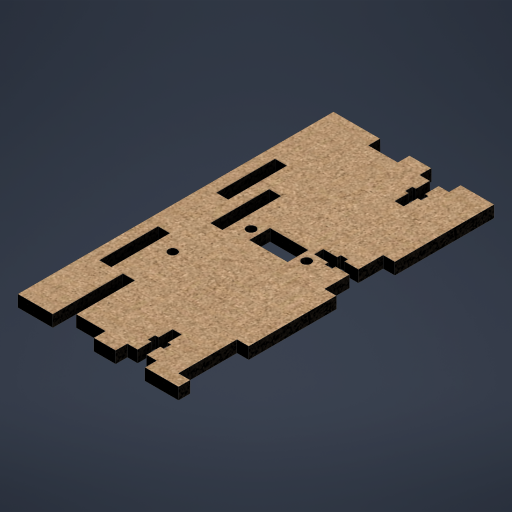
# Autodesk Inventor part: FloorButtonHolder_Top_V1_B
Saved by Autodesk Inventor 2024.1 (Build 281209000, 209)
## iProperties
Created: 2023-05-20
Part Number: FloorButtonHolder_Top_V1_B
Material: MDF Medium Density Fiberboard
Document SubType Name: Modeling
Designer: jaege
Density: 0.8 g/cm^3
Appearance: Cardboard - Corrugated
Author: jaege
Autodesk Inventor part; units mm, degrees
ref_plane "YZ Plane" through (0, 0, 0) normal (1, 0, 0) x (0, 1, 0)
ref_plane "XZ Plane" through (0, 0, 0) normal (0, 1, 0) x (-1, 0, 0)
ref_plane "XY Plane" through (0, 0, 0) normal (0, 0, 1) x (1, 0, 0)
sketch "Sketch1" plane through (0, 0, 0) normal (0, 1, 0) x (-1, 0, 0)
  line L0 (-17.5, 50) -> (17.5, 50)
  line L1 (17.5, 50) -> (17.5, -50)
  line L2 (17.5, -50) -> (-17.5, -50)
  line L3 (-17.5, -50) -> (-17.5, 50)
  line L4 (-17.5, 50) -> (17.5, -50) construction
  line L5 (17.5, 50) -> (-17.5, -50) construction
  line L6 (7.5, 50) -> (0, 50)
  line L7 (0, 50) -> (0, 54)
  line L8 (0, 54) -> (7.5, 54)
  line L9 (7.5, 54) -> (7.5, 50)
  line L10 (-10, 50) -> (-21.5, 50)
  line L11 (-21.5, 50) -> (-21.5, 54)
  line L12 (-21.5, 54) -> (-10, 54)
  line L13 (-10, 54) -> (-10, 50)
  line L14 (17.5, 30) -> (21.5, 30)
  line L15 (21.5, 30) -> (21.5, 0)
  line L16 (21.5, 0) -> (17.5, 0)
  line L17 (17.5, 0) -> (17.5, 30)
  line L18 (17.5, -20) -> (21.5, -20)
  line L19 (21.5, -20) -> (21.5, -54)
  line L20 (21.5, -54) -> (17.5, -54)
  line L21 (17.5, -54) -> (17.5, -20)
  line L22 (7.5, -50) -> (0, -50)
  line L23 (0, -50) -> (0, -54)
  line L24 (0, -54) -> (7.5, -54)
  line L25 (7.5, -54) -> (7.5, -50)
  line L26 (-10, -50) -> (-21.5, -50)
  line L27 (-21.5, -50) -> (-21.5, -54)
  line L28 (-21.5, -54) -> (-10, -54)
  line L29 (-10, -54) -> (-10, -50)
  line L30 (-17.5, 30) -> (-21.5, 30)
  line L31 (-21.5, 30) -> (-21.5, 0)
  line L32 (-21.5, 0) -> (-17.5, 0)
  line L33 (-17.5, 0) -> (-17.5, 30)
  line L34 (-17.5, -50) -> (-21.5, -50)
  line L35 (-21.5, -50) -> (-21.5, -20)
  line L36 (-21.5, -20) -> (-17.5, -20)
  line L37 (-17.5, -20) -> (-17.5, -50)
  point P0 (0, 0)
  point P1 (17.5, 0)
  point P2 (-17.5, 0)
  point P3 (-17.5, -20)
  point P4 (-21.5, -50)
  point P5 (0, -50)
  point P6 (17.5, -50)
  dimension "d0" = 35
  dimension "d2" = 7.5
  dimension "d3" = 4
  dimension "d4" = 11.5
  dimension "d5" = 4
  dimension "d6" = 10
  dimension "d7" = 10
  dimension "d8" = 4
  dimension "d9" = 30
  dimension "d10" = 4
  dimension "d11" = 34
  dimension "d12" = 20
  dimension "d13" = 20
  dimension "d14" = 7.5
  dimension "d15" = 4
  dimension "d16" = 11.5
  dimension "d17" = 4
  dimension "d18" = 10
  dimension "d19" = 10
  dimension "d20" = 4
  dimension "d21" = 30
  dimension "d22" = 20
  dimension "d23" = 4
  dimension "d24" = 30
  dimension "d27" = 4
  constraints: 76 end point, 18 parallel, 9 horizontal, 9 perpendicular, 7 point on line, 2 midpoint
  measures "d0" distance of L1.end L2.end
  measures "d2" distance of L7.end L8.end
  measures "d3" distance of L6.end L7.end
  measures "d4" distance of L11.end L12.end
  measures "d5" distance of L10.end L11.end
  measures "d6" distance between parallel lines of L9 L1
  measures "d7" distance between parallel lines of L13 L7
  measures "d8" distance of L15.end L16.end
  measures "d9" distance of L14.end L15.end
  measures "d10" distance of L19.end L20.end
  measures "d11" distance of L18.end L19.end
  measures "d12" distance between parallel lines of L16 L18
  measures "d13" distance between parallel lines of L0 L14
  measures "d14" distance of L24.end L23.end
  measures "d15" distance of L23.end L22.end
  measures "d16" distance of L28.end L27.end
  measures "d17" distance of L27.end L26.end
  measures "d18" distance between parallel lines of L25 L21
  measures "d19" distance between parallel lines of L29 L23
  measures "d20" distance of L32.end L31.end
  measures "d21" distance of L31.end L30.end
  measures "d22" distance between parallel lines of L10 L30
  measures "d23" distance of L35.end L36.end
  measures "d24" distance of L34.end L35.end
  measures "d27" distance between parallel lines of L2 L20
extrude "Extrusion1" add sketch "Sketch1" along normal blind 4
sketch "Sketch2" plane through (0, 4, 0) normal (0, 1, 0) x (1, 0, 0)
  line L0 (-21.5, 54) -> (-33.5, 54)
  line L1 (-33.5, 54) -> (-33.5, -54)
  line L2 (-33.5, -54) -> (-21.5, -54)
  line L3 (-21.5, -54) -> (-21.5, 54)
  line L4 (-7.5, -54) -> (0, -54) projected
  line L5 (-21.5, 54) -> (-21.5, 20) projected
  line L6 (-21.5, 20) -> (-17.5, 20) projected
  line L7 (-17.5, 20) -> (-17.5, 0) projected
  line L8 (-17.5, 0) -> (-21.5, 0) projected
  line L9 (-21.5, 0) -> (-21.5, -30) projected
  line L10 (-21.5, -30) -> (-17.5, -30) projected
  line L11 (-17.5, -30) -> (-17.5, -50) projected
  line L12 (-17.5, -50) -> (-7.5, -50) projected
  line L13 (-7.5, -50) -> (-7.5, -54) projected
  line L14 (-7.5, -54) -> (0, -54) projected
  line L15 (0, -54) -> (0, -50) projected
  line L16 (0, -50) -> (10, -50) projected
  line L17 (10, -50) -> (10, -54) projected
  line L18 (10, -54) -> (21.5, -54) projected
  line L19 (21.5, -54) -> (21.5, -50) projected
  line L20 (21.5, -50) -> (17.5, -50) projected
  line L21 (17.5, -50) -> (17.5, -30) projected
  line L22 (17.5, -30) -> (21.5, -30) projected
  line L23 (21.5, -30) -> (21.5, 0) projected
  line L24 (21.5, 0) -> (17.5, 0) projected
  line L25 (17.5, 0) -> (17.5, 20) projected
  line L26 (17.5, 20) -> (21.5, 20) projected
  line L27 (21.5, 20) -> (21.5, 54) projected
  line L28 (21.5, 54) -> (10, 54) projected
  line L29 (10, 54) -> (10, 50) projected
  line L30 (10, 50) -> (0, 50) projected
  line L31 (0, 50) -> (0, 54) projected
  line L32 (0, 54) -> (-7.5, 54) projected
  line L33 (-7.5, 54) -> (-7.5, 50) projected
  line L34 (-7.5, 50) -> (-17.5, 50) projected
  line L35 (-17.5, 50) -> (-17.5, 54) projected
  line L36 (-17.5, 54) -> (-21.5, 54) projected
  line L37 (-29.5, 30) -> (-25.5, 30)
  line L38 (-25.5, 30) -> (-25.5, 10)
  line L39 (-25.5, 10) -> (-29.5, 10)
  line L40 (-29.5, 10) -> (-29.5, 30)
  line L41 (-25.5, -30) -> (-29.5, -30)
  line L42 (-29.5, -30) -> (-29.5, -10)
  line L43 (-29.5, -10) -> (-25.5, -10)
  line L44 (-25.5, -10) -> (-25.5, -30)
  line L45 (-29.5, 10) -> (-25.5, -10) construction
  point P0 (0, 0)
  point P1 (-27.5, 0)
  point P2 (-33.5, 0)
  dimension "d29" = 4
  dimension "d30" = 20
  dimension "d31" = 20
  dimension "d32" = 4
  dimension "d35" = 51
  constraints: 26 end point, 6 parallel, 3 horizontal, 3 perpendicular, 2 equal length, 2 midpoint, 1 coincident, 1 collinear, 1 horizontal alignment, 1 vertical alignment
  measures "d29" distance of L37.start L37.end
  measures "d30" distance of L37.end L38.end
  measures "d31" distance between parallel lines of L43 L39
  measures "d32" distance between parallel lines of L1 L40
  measures "d35" distance between parallel lines of L25 L1
extrude "Extrusion2" add sketch "Sketch2" against normal up to surface (4 mm away) contours L3 L2 L1 L0
sketch "Sketch3" plane through (0, 4, 0) normal (0, 1, 0) x (1, 0, 0)
  line L0 (-1.8, 2) -> (-1.8, 8.3) construction
  line L1 (17.5, 0) -> (17.5, 20) projected
  line L2 (-21.5, -30) -> (-17.5, -30) projected
  line L3 (-17.5, -30) -> (-17.5, -50) projected
  line L4 (-17.5, -50) -> (-7.5, -50) projected
  line L5 (-7.5, -50) -> (-7.5, -54) projected
  line L6 (-7.5, -54) -> (0, -54) projected
  line L7 (0, -54) -> (0, -50) projected
  line L8 (0, -50) -> (10, -50) projected
  line L9 (10, -50) -> (10, -54) projected
  line L10 (10, -54) -> (21.5, -54) projected
  line L11 (21.5, -54) -> (21.5, -50) projected
  line L12 (21.5, -50) -> (17.5, -50) projected
  line L13 (17.5, -50) -> (17.5, -30) projected
  line L14 (17.5, -30) -> (21.5, -30) projected
  line L15 (21.5, -30) -> (21.5, 0) projected
  line L16 (21.5, 0) -> (17.5, 0) projected
  line L17 (17.5, 0) -> (17.5, 20) projected
  line L18 (17.5, 20) -> (21.5, 20) projected
  line L19 (21.5, 20) -> (21.5, 54) projected
  line L20 (21.5, 54) -> (10, 54) projected
  line L21 (10, 54) -> (10, 50) projected
  line L22 (10, 50) -> (0, 50) projected
  line L23 (0, 50) -> (0, 54) projected
  line L24 (0, 54) -> (-7.5, 54) projected
  line L25 (-7.5, 54) -> (-7.5, 50) projected
  line L26 (-7.5, 50) -> (-17.5, 50) projected
  line L27 (-17.5, 50) -> (-17.5, 54) projected
  line L28 (-17.5, 54) -> (-33.5, 54) projected
  line L29 (-33.5, 54) -> (-33.5, -54) projected
  line L30 (-33.5, -54) -> (-21.5, -54) projected
  line L31 (-21.5, -54) -> (-21.5, -30) projected
  line L32 (-25.5, -30) -> (-29.5, -30) projected
  line L33 (-29.5, -30) -> (-29.5, -10) projected
  line L34 (-29.5, -10) -> (-25.5, -10) projected
  line L35 (-25.5, -10) -> (-25.5, -30) projected
  line L36 (-29.5, 30) -> (-25.5, 30) projected
  line L37 (-25.5, 30) -> (-25.5, 10) projected
  line L38 (-25.5, 10) -> (-29.5, 10) projected
  line L39 (-29.5, 10) -> (-29.5, 30) projected
  line L40 (-21.5, 0) -> (-21.5, 20) projected
  line L41 (-21.5, 20) -> (-17.5, 20) projected
  line L42 (-17.5, 20) -> (-17.5, 0) projected
  line L43 (-17.5, 0) -> (-21.5, 0) projected
  line L44 (-25.5, 10) -> (-29.5, 10) projected
  line L45 (-25.5, -30) -> (-25.5, -10) projected
  line L46 (-29.5, 10) -> (-25.5, -10) construction
  point P0 (0, 0)
  point P1 (-27.5, 0)
  point P2 (6.15, 5.15)
  point P3 (-12.85, 5.15)
  point P4 (-1.8, 5.15)
  dimension "d36" = 19.3
  dimension "d37" = 6.3
  dimension "d38" = 2
  dimension "d39" = 7.95
  dimension "d40" = 11.05
  constraints: 4 end point, 2 horizontal alignment, 2 midpoint
  measures "d36" distance between parallel lines of L1 L0
  measures "d37" distance of L0.start L0.end
  measures "d38" vertical distance of L0.start point (-27.5, 0)
  measures "d39" distance from line of point (6.15, 5.15) L0
  measures "d40" distance from line of L0 point (-12.85, 5.15)
hole "Hole1" at (-12.85, 4, -5.15) at (6.15, 4, -5.15) direction (0, -1, 0) diameter 3.1 depth 4
sketch "Sketch4" plane through (0, 4, 0) normal (0, 1, 0) x (1, 0, 0)
  circle A0 centre (-12.85, 5.15) radius 1.55 projected
  circle A1 centre (6.15, 5.15) radius 1.55 projected
  line L0 (-21.5, -30) -> (-17.5, -30) projected
  line L1 (-17.5, -30) -> (-17.5, -50) projected
  line L2 (-17.5, -50) -> (-7.5, -50) projected
  line L3 (-7.5, -50) -> (-7.5, -54) projected
  line L4 (-7.5, -54) -> (0, -54) projected
  line L5 (0, -54) -> (0, -50) projected
  line L6 (0, -50) -> (10, -50) projected
  line L7 (10, -50) -> (10, -54) projected
  line L8 (10, -54) -> (21.5, -54) projected
  line L9 (21.5, -54) -> (21.5, -50) projected
  line L10 (21.5, -50) -> (17.5, -50) projected
  line L11 (17.5, -50) -> (17.5, -30) projected
  line L12 (17.5, -30) -> (21.5, -30) projected
  line L13 (21.5, -30) -> (21.5, 0) projected
  line L14 (21.5, 0) -> (17.5, 0) projected
  line L15 (17.5, 0) -> (17.5, 20) projected
  line L16 (17.5, 20) -> (21.5, 20) projected
  line L17 (21.5, 20) -> (21.5, 54) projected
  line L18 (21.5, 54) -> (10, 54) projected
  line L19 (10, 54) -> (10, 50) projected
  line L20 (10, 50) -> (0, 50) projected
  line L21 (0, 50) -> (0, 54) projected
  line L22 (0, 54) -> (-7.5, 54) projected
  line L23 (-7.5, 54) -> (-7.5, 50) projected
  line L24 (-7.5, 50) -> (-17.5, 50) projected
  line L25 (-17.5, 50) -> (-17.5, 54) projected
  line L26 (-17.5, 54) -> (-33.5, 54) projected
  line L27 (-33.5, 54) -> (-33.5, -54) projected
  line L28 (-33.5, -54) -> (-21.5, -54) projected
  line L29 (-21.5, -54) -> (-21.5, -30) projected
  line L30 (-25.5, -30) -> (-29.5, -30) projected
  line L31 (-29.5, -30) -> (-29.5, -10) projected
  line L32 (-29.5, -10) -> (-25.5, -10) projected
  line L33 (-25.5, -10) -> (-25.5, -30) projected
  line L34 (-29.5, 30) -> (-25.5, 30) projected
  line L35 (-25.5, 30) -> (-25.5, 10) projected
  line L36 (-25.5, 10) -> (-29.5, 10) projected
  line L37 (-29.5, 10) -> (-29.5, 30) projected
  line L38 (-21.5, 0) -> (-21.5, 20) projected
  line L39 (-21.5, 20) -> (-17.5, 20) projected
  line L40 (-17.5, 20) -> (-17.5, 0) projected
  line L41 (-17.5, 0) -> (-21.5, 0) projected
  line L42 (-9.85, 8.65) -> (3.15, 8.65)
  line L43 (3.15, 8.65) -> (3.15, 1.65)
  line L44 (3.15, 1.65) -> (-9.85, 1.65)
  line L45 (-9.85, 1.65) -> (-9.85, 8.65)
  line L46 (-12.85, 5.15) -> (-9.85, 5.15) construction
  line L47 (3.15, 5.15) -> (6.15, 5.15) construction
  point P0 (0, 0)
  dimension "d49" = 7
  dimension "d54" = 3
  constraints: 12 end point, 3 equal length, 2 horizontal, 2 midpoint, 1 collinear, 1 horizontal alignment, 1 perpendicular
  measures "d49" distance of L42.end L43.end
  measures "d54" distance from line of L46.start L45
extrude "Extrusion3" cut sketch "Sketch4" against normal through all contours L42 L43 L44 L45
sketch "Sketch5" plane through (0, 4, 0) normal (0, 1, 0) x (1, 0, 0)
  line L0 (12.7, 11.5) -> (17.5, 11.5) projected
  line L1 (17.5, 11.5) -> (17.5, 20) construction
  line L2 (17.5, 20) -> (21.5, 20) construction
  line L3 (21.5, 20) -> (21.5, 54) construction
  line L4 (21.5, 54) -> (10, 54) construction
  line L5 (10, 54) -> (10, 50) construction
  line L6 (10, 50) -> (6.5, 50) construction
  line L7 (6.5, 50) -> (6.5, 45.2) projected
  line L8 (6.5, 45.2) -> (7.7, 45.2) projected
  line L9 (7.7, 45.2) -> (7.7, 42.8) projected
  line L10 (7.7, 42.8) -> (6.5, 42.8) projected
  line L11 (6.5, 42.8) -> (6.5, 38) projected
  line L12 (6.5, 38) -> (3.5, 38) projected
  line L13 (3.5, 38) -> (3.5, 42.8) projected
  line L14 (3.5, 42.8) -> (2.3, 42.8) projected
  line L15 (2.3, 42.8) -> (2.3, 45.2) projected
  line L16 (2.3, 45.2) -> (3.5, 45.2) projected
  line L17 (3.5, 45.2) -> (3.5, 50) projected
  line L18 (3.5, 50) -> (0, 50) construction
  line L19 (0, 50) -> (0, 54) construction
  line L20 (0, 54) -> (-7.5, 54) construction
  line L21 (-7.5, 54) -> (-7.5, 50) construction
  line L22 (-7.5, 50) -> (-17.5, 50) construction
  line L23 (-17.5, 50) -> (-17.5, 54) construction
  line L24 (-17.5, 54) -> (-33.5, 54) construction
  line L25 (-33.5, 54) -> (-33.5, -54) construction
  line L26 (-33.5, -54) -> (-21.5, -54) construction
  line L27 (-21.5, -54) -> (-21.5, -30) construction
  line L28 (-21.5, -30) -> (-17.5, -30) construction
  line L29 (-17.5, -30) -> (-17.5, -50) construction
  line L30 (-17.5, -50) -> (-7.5, -50) construction
  line L31 (-7.5, -50) -> (-7.5, -54) construction
  line L32 (-7.5, -54) -> (0, -54) construction
  line L33 (0, -54) -> (0, -50) projected
  line L34 (0, -50) -> (3.5, -50) projected
  line L35 (3.5, -50) -> (3.5, -45.2) projected
  line L36 (3.5, -45.2) -> (2.3, -45.2) projected
  line L37 (2.3, -45.2) -> (2.3, -42.8) projected
  line L38 (2.3, -42.8) -> (3.5, -42.8) projected
  line L39 (3.5, -42.8) -> (3.5, -38) projected
  line L40 (3.5, -38) -> (6.5, -38) projected
  line L41 (6.5, -38) -> (6.5, -42.8) projected
  line L42 (6.5, -42.8) -> (7.7, -42.8) projected
  line L43 (7.7, -42.8) -> (7.7, -45.2) projected
  line L44 (7.7, -45.2) -> (6.5, -45.2) projected
  line L45 (6.5, -45.2) -> (6.5, -50) projected
  line L46 (6.5, -50) -> (10, -50) construction
  line L47 (10, -50) -> (10, -54) construction
  line L48 (10, -54) -> (21.5, -54) construction
  line L49 (21.5, -54) -> (21.5, -50) construction
  line L50 (21.5, -50) -> (17.5, -50) construction
  line L51 (17.5, -50) -> (17.5, -30) construction
  line L52 (17.5, -30) -> (21.5, -30) construction
  line L53 (21.5, 0) -> (17.5, 0) construction
  line L54 (17.5, 0) -> (17.5, 8.5) construction
  line L55 (17.5, 8.5) -> (12.7, 8.5) projected
  line L56 (12.7, 8.5) -> (12.7, 7.3) projected
  line L57 (12.7, 7.3) -> (10.3, 7.3) projected
  line L58 (10.3, 7.3) -> (10.3, 8.5) projected
  line L59 (10.3, 8.5) -> (5.5, 8.5) projected
  line L60 (5.5, 8.5) -> (5.5, 11.5) projected
  line L61 (5.5, 11.5) -> (10.3, 11.5) projected
  line L62 (10.3, 11.5) -> (10.3, 12.7) projected
  line L63 (10.3, 12.7) -> (12.7, 12.7) projected
  line L64 (12.7, 12.7) -> (12.7, 11.5) projected
  circle A0 centre (-19.5, -15) radius 1.5 projected
  line L65 (-29.5, 10) -> (-25.5, 10) construction
  line L66 (-25.5, 10) -> (-25.5, -10) construction
  line L67 (-25.5, -10) -> (-29.5, -10) construction
  line L68 (-29.5, -10) -> (-29.5, 10) construction
  line L69 (-21.5, 0) -> (-21.5, 20) construction
  line L70 (-21.5, 20) -> (-17.5, 20) construction
  line L71 (-17.5, 20) -> (-17.5, 0) construction
  line L72 (-17.5, 0) -> (-21.5, 0) construction
  line L73 (3.5, 50) -> (6.5, 50)
  line L74 (10, 50) -> (0, 50) projected
  line L75 (17.5, 11.5) -> (17.5, 8.5)
  line L76 (3.5, -50) -> (6.5, -50)
  line L77 (0, -50) -> (10, -50) projected
  point P0 (0, 0)
  constraints: 6 end point, 2 collinear, 1 perpendicular
extrude "Extrusion4" cut sketch "Sketch5" against normal up to next
body "Solid1"
